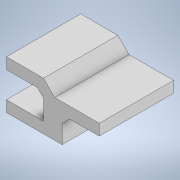
# Autodesk Inventor part: test_support2
Saved by Autodesk Inventor 2020 (Build 240168000, 168)
## iProperties
Created: 2024-02-14
Part Number: test_support2
Material: Типовые
Document SubType Name: Modeling
Designer: 4s
Density: 1 g/cm^3
Appearance: По умолчанию
Author: 4s
Autodesk Inventor part; units mm, degrees
ref_plane "YZ Plane" through (0, 0, 0) normal (1, 0, 0) x (0, 1, 0)
ref_plane "XZ Plane" through (0, 0, 0) normal (0, 1, 0) x (-1, 0, 0)
ref_plane "XY Plane" through (0, 0, 0) normal (0, 0, 1) x (1, 0, 0)
sketch "Эскиз1" plane through (0, 0, 0) normal (0, 1, 0) x (-1, 0, 0)
  line L0 (0, 0) -> (-5, 0)
  line L1 (-5, 0) -> (-5, -20)
  line L2 (-5, -20) -> (0, -20)
  line L3 (0, -20) -> (0, 0)
  dimension "d0" = 5
  dimension "d1" = 20
  constraints: 8 end point, 2 parallel, 1 horizontal, 1 perpendicular
  measures "d0" distance of L2.end L1.end
  measures "d1" distance of L1.end L0.end
extrude "Выдавливание1" add sketch "Эскиз1" along normal blind 7
sketch "Эскиз2" plane through (0, 7, 0) normal (0, 1, 0) x (1, 0, 0)
  line L0 (0, 0) -> (5, 0) projected
  line L1 (5, 0) -> (5, 20) projected
  line L2 (5, 20) -> (0, 20) projected
  line L3 (0, 20) -> (0, 0) projected
  line L4 (0, 0) -> (5, 0) projected
  line L5 (5, 0) -> (15, 0)
  line L6 (15, 0) -> (15, 20)
  line L7 (15, 20) -> (5, 20)
  line L8 (5, 20) -> (5, 0)
  dimension "d4" = 10
  dimension "d5" = 20
  constraints: 8 end point, 2 parallel, 1 horizontal, 1 perpendicular
  measures "d4" distance of L7.end L6.end
  measures "d5" distance of L6.end L5.end
extrude "Выдавливание2" add sketch "Эскиз2" along normal blind 3
chamfer "Фаска1" distance 2 angle 45 1 edges at (5, 7, -10)
sketch "Эскиз3" plane through (0, 0, 0) normal (0, 0, 1) x (1, 0, 0)
  line L0 (0, 0) -> (25, 0)
  line L1 (25, 0) -> (25, 3)
  line L2 (25, 3) -> (0, 3)
  line L3 (0, 3) -> (0, 0)
  line L4 (0, 0) -> (5, 0) construction
  line L5 (5, 0) -> (5, 5) construction
  line L6 (7, 7) -> (5, 5) construction
  line L7 (7, 7) -> (15, 7) construction
  line L8 (15, 7) -> (15, 10) construction
  line L9 (0, 10) -> (15, 10) construction
  line L10 (0, 0) -> (0, 10) construction
  line L11 (0, 3) -> (5, 3)
  line L12 (5, 3) -> (5, 13)
  line L13 (5, 13) -> (0, 13)
  line L14 (0, 13) -> (0, 3)
  line L15 (5, 13) -> (15, 13)
  line L16 (15, 13) -> (15, 10)
  line L17 (15, 10) -> (5, 10)
  line L18 (5, 10) -> (5, 13)
  line L19 (0, 0) -> (5, 0) projected
  line L20 (0, 0) -> (-10, 0)
  line L21 (-10, 0) -> (-10, 3)
  line L22 (-10, 3) -> (0, 3)
  line L23 (0, 3) -> (0, 0)
  line L24 (0, 13) -> (-10, 13)
  line L25 (-10, 13) -> (-10, 10)
  line L26 (-10, 10) -> (0, 10)
  line L27 (0, 10) -> (0, 13)
  line L28 (0, 13) -> (3, 10)
  line L29 (0, 10) -> (15, 10) projected
  line L30 (-1.6585, 10) -> (0, 8.3415)
  line L31 (0, 0) -> (0, 10) projected
  point P0 (0, 8.3415)
  dimension "d11" = 3
  dimension "d12" = 25
  dimension "d13" = 5
  dimension "d14" = 10
  dimension "d15" = 10
  dimension "d16" = 3
  dimension "d17" = 10
  dimension "d18" = 3
  constraints: 44 end point, 10 parallel, 5 horizontal, 5 perpendicular, 2 point on line, 2 other
  measures "d11" distance of L1.end L0.end
  measures "d12" distance of L0.start L0.end
  measures "d13" distance of L13.end L12.end
  measures "d14" distance of L12.end L11.end
  measures "d15" distance of L21.end L22.end
  measures "d16" distance of L20.end L21.end
  measures "d17" distance of L26.end L25.end
  measures "d18" distance of L25.end L24.end
extrude "Выдавливание3" add sketch "Эскиз3" against normal blind 20 contours L20 L21 L22 L3 | L30 L26 L14 | L26 L25 L24 L14 | L14 L28 L29
